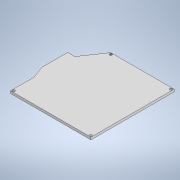
# Autodesk Inventor part: CaseCover
Saved by Autodesk Inventor 2020.1 (Build 241239000, 239)
## iProperties
Created: 2020-05-23
Part Number: CaseCover
Material: Generic
Document SubType Name: Modeling
Designer: super
Density: 1 g/cm^3
Appearance: Default
Author: super
Autodesk Inventor part; units mm, degrees
ref_plane "YZ Plane" through (0, 0, 0) normal (1, 0, 0) x (0, 1, 0)
ref_plane "XZ Plane" through (0, 0, 0) normal (0, 1, 0) x (-1, 0, 0)
ref_plane "XY Plane" through (0, 0, 0) normal (0, 0, 1) x (1, 0, 0)
sketch "Sketch1" plane through (0, 0, 0) normal (0, 1, 0) x (-1, 0, 0)
  line L0 (0, 0) -> (0, -51.9)
  line L1 (0, -51.9) -> (39.53, -51.9)
  line L2 (0, 0) -> (53.1, 0)
  line L3 (0, 0) -> (50.2, 0)
  line L4 (50.2, 0) -> (50.2, -14.6)
  line L5 (50.2, 0) -> (64.8, 0) construction
  line L6 (50.2, -14.6) -> (53.1008, -22.6003)
  line L7 (50.2, -14.6) -> (58.71, -14.6) construction
  line L8 (53.1008, -22.6003) -> (53.1008, -38.4903)
  line L9 (53.1008, -38.4903) -> (48.6508, -38.4903)
  line L10 (48.6508, -38.4903) -> (39.53, -51.9)
  dimension "d0" = 51.9
  dimension "d1" = 39.53
  dimension "d9" = 50.2
  dimension "d10" = 14.6
  dimension "d11" = 90
  dimension "d12" = 8.51
  dimension "d13" = 70.07
  dimension "d14" = 15.89
  dimension "d17" = 4.45
  constraints: 22 end point, 4 horizontal, 3 vertical, 2 equal length, 1 perpendicular, 1 point on line
  measures "d0" distance of L0.start L0.end
  measures "d1" distance of L0.end L1.end
  measures "d9" distance of L0.start L3.end
  measures "d10" distance of L3.end L4.end
  measures "d11" angle of L4 L5
  measures "d12" distance of L4.end L6.end
  measures "d13" angle of L6 L7
  measures "d14" distance of L6.end L8.end
  measures "d17" distance of L8.end L9.end
extrude "Extrusion1" add sketch "Sketch1" along normal blind 1.5
sketch "Sketch2" plane through (0, 1.5, 0) normal (0, 1, 0) x (1, 0, 0)
  circle A0 centre (-1, 1) radius 0.75
  point P0 (0, 0)
  dimension "d22" = 1.5
  constraints: 1 centre point
  measures "d22" diameter of A0
extrude "Extrusion2" cut sketch "Sketch2" against normal blind 10
sketch "Sketch3" plane through (0, 1.5, 0) normal (0, 1, 0) x (1, 0, 0)
  line L0 (0, 0) -> (0, 51.9) projected
  line L1 (0, 51.9) -> (-39.53, 51.9) projected
  circle A0 centre (-1, 50.9) radius 0.75
  dimension "d27" = 1.5
  constraints: 1 centre point
  measures "d27" diameter of A0
extrude "Extrusion3" cut sketch "Sketch3" against normal blind 10
sketch "Sketch4" plane through (0, 1.5, 0) normal (0, 1, 0) x (1, 0, 0)
  circle A0 centre (-49.2, 1) radius 0.75
  line L0 (-39.53, 51.9) -> (-48.6508, 38.4903) projected
  circle A1 centre (-38.53, 50.9) radius 0.75
  point P0 (0, 0)
  point P1 (-50.2, 0)
  dimension "d32" = 1.5
  dimension "d35" = 1.5
  constraints: 2 centre point
  measures "d32" diameter of A0
  measures "d35" diameter of A1
extrude "Extrusion4" cut sketch "Sketch4" against normal blind 10
body "Solid1"
